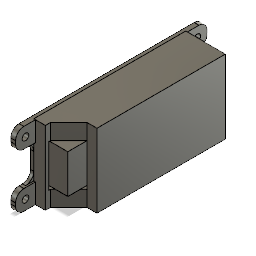
Kanssi_v2 (Autodesk Fusion 360 design; units mm, degrees)
Autodesk Fusion 360 part; units mm, degrees
sketch "PCB" plane through (0, 0, 0) normal (1, 0, 0) x (0, 0, -1)
  line L0 (0, 0) -> (-84.582, 0)
  line L1 (-84.582, 0) -> (-84.582, 37.465)
  line L2 (-84.582, 37.465) -> (0, 37.465)
  line L3 (0, 37.465) -> (0, 0)
  circle A0 centre (-78.867, 3.175) radius 1.55
  circle A1 centre (-3.683, 3.175) radius 1.55
  circle A2 centre (-78.867, 34.29) radius 1.55
  circle A3 centre (-3.683, 34.29) radius 1.55
  dimension "d1" = 37.465
  dimension "d2" = 84.582
  dimension "d3" = 3.1
  dimension "d4" = 75.184
  dimension "d5" = 3.1
  dimension "d7" = 31.115
  dimension "d10" = 5.715
  dimension "d11" = 3.175
  dimension "d12" = 3.1
  dimension "d242" = 3.1
  constraint horizontal L0
  constraint vertical L1
  constraint horizontal L2
  constraint vertical L3
  constraint coincident L0.start L3.end
  measures "d1" distance of L0.start L2.end
  measures "d2" distance of L0.start L0.end
  measures "d3" diameter of A1
  measures "d4" distance of A0.centre A1.centre
  measures "d5" diameter of A2
  measures "d7" distance of A0.centre A2.centre
  measures "d10" distance of L1 A0.centre
  measures "d11" distance of L0 A0.centre
  measures "d12" diameter of A3
  measures "d242" diameter of A0
extrude "Extrude1" add sketch "PCB" along normal blind 2 makes body 1
sketch "Komponentit" plane through (2, 0, 0) normal (1, 0, 0) x (0, 0, -1)
  circle A0 centre (-3.683, 3.175) radius 1.55
  circle A1 centre (-78.867, 34.29) radius 1.55
  circle A2 centre (-78.867, 3.175) radius 1.55
  circle A3 centre (-3.683, 34.29) radius 1.55
  line L0 (0, 37.465) -> (-84.582, 37.465)
  line L1 (-84.582, 37.465) -> (-84.582, 0)
  line L2 (-84.582, 0) -> (0, 0)
  line L3 (0, 0) -> (0, 37.465)
  line L4 (-44.958, 11.557) -> (-70.358, 11.557)
  line L5 (-70.358, 36.957) -> (-44.958, 36.957)
  line L6 (-70.358, 36.957) -> (-44.958, 36.957)
  line L7 (-44.958, 36.957) -> (-44.958, 11.557)
  line L8 (-44.958, 11.557) -> (-70.358, 11.557)
  line L9 (-70.358, 11.557) -> (-70.358, 36.957)
  line L10 (-84.582, 37.465) -> (0, 37.465)
  line L11 (0, 37.465) -> (0, 0)
  line L12 (0, 0) -> (-84.582, 0)
  line L13 (-84.582, 0) -> (-84.582, 37.465)
  line L14 (-70.358, 11.1514) -> (-44.9504, 11.1514)
  line L15 (-44.9504, 11.1514) -> (-44.9504, 0.635)
  line L16 (-44.9504, 0.635) -> (-70.358, 0.635)
  line L17 (-70.358, 0.635) -> (-70.358, 11.1514)
  line L18 (-44.5991, 24) -> (-22.6991, 24)
  line L19 (-22.6991, 24) -> (-22.6991, 1.1)
  line L20 (-22.6991, 1.1) -> (-44.5991, 1.1)
  line L21 (-44.5991, 1.1) -> (-44.5991, 24)
  line L22 (-84.582, 30.48) -> (-71, 30.48)
  line L23 (-71, 30.48) -> (-71, 7.112)
  line L24 (-71, 7.112) -> (-84.582, 7.112)
  line L25 (-84.582, 7.112) -> (-84.582, 30.48)
  line L26 (0, 37.465) -> (-28, 37.465)
  line L27 (0, 37.465) -> (-21, 37.465)
  line L28 (-28, 37.465) -> (-21, 37.465)
  line L29 (-21, 37.465) -> (-21, 26.465)
  line L30 (-21, 26.465) -> (-28, 26.465)
  line L31 (-28, 26.465) -> (-28, 37.465)
  dimension "d22" = 25.4
  dimension "d23" = 14.224
  dimension "d24" = 0.508
  dimension "d25" = 25.4
  dimension "d26" = 10.5164
  dimension "d27" = 25.4076
  dimension "d28" = 0.635
  dimension "d29" = 14.224
  dimension "d30" = 21.9
  dimension "d31" = 22.9
  dimension "d33" = 1.1
  dimension "d34" = 0.3589
  dimension "d41" = 7.112
  dimension "d42" = 6.985
  dimension "d43" = 0.642
  dimension "d355" = 28
  dimension "d356" = 21
  dimension "d357" = 11
  constraint horizontal L4
  constraint horizontal L6
  constraint vertical L7
  constraint horizontal L8
  constraint vertical L9
  constraint horizontal L10
  constraint vertical L11
  constraint horizontal L12
  constraint vertical L13
  constraint coincident L2.end L3.start
  constraint coincident L0.end L1.start
  constraint horizontal L14
  constraint vertical L15
  constraint horizontal L16
  constraint vertical L17
  constraint horizontal L18
  constraint vertical L19
  constraint horizontal L20
  constraint vertical L21
  constraint horizontal L22
  constraint vertical L23
  constraint horizontal L24
  constraint vertical L25
  constraint coincident L1 L22.start
  constraint coincident L0.start L3.end
  constraint perpendicular L3 L26
  constraint perpendicular L11 L27
  constraint horizontal L28
  constraint vertical L29
  constraint horizontal L30
  constraint vertical L31
  measures "d22" distance of L4 L5
  measures "d23" distance of L9 L13
  measures "d24" distance of L6 L10
  measures "d25" distance of L7 L9
  measures "d26" distance of L14.start L16.end
  measures "d27" distance of L15 L17
  measures "d28" distance of L12 L16
  measures "d29" distance of L13 L17
  measures "d30" distance of L19 L21
  measures "d31" distance of L18 L20
  measures "d33" distance of L12 L20
  measures "d34" distance of L7 L21
  measures "d41" distance of L12 L24
  measures "d42" distance of L10 L22
  measures "d43" distance of L9 L23
  measures "d355" distance of L0.start L26.end
  measures "d356" distance of L0.start L27.end
  measures "d357" distance of L26.end L30.end
extrude "Extrude4" add sketch "Komponentit" along normal blind 15 contours L18 L19 L20 L21 bodies 1
extrude "Extrude3" add sketch "Komponentit" along normal blind 15.8 contours L14 L15 L16 L17 bodies 1
extrude "Extrude2" add sketch "Komponentit" along normal blind 16.3 contours L4 L5 L6 L7 L8 L9 bodies 1
sketch "Sketch7" plane through (2, 0, 0) normal (1, 0, 0) x (0, 0, -1)
  line L0 (-70.358, 11.557) -> (-70.358, 36.957)
  line L1 (-70.358, 36.957) -> (-44.958, 36.957)
  line L2 (-44.958, 36.957) -> (-44.958, 11.557)
  line L3 (-44.958, 11.557) -> (-70.358, 11.557)
  line L4 (-70.358, 0.635) -> (-70.358, 11.1514)
  line L5 (-70.358, 11.1514) -> (-44.9504, 11.1514)
  line L6 (-44.9504, 11.1514) -> (-44.9504, 0.635)
  line L7 (-44.9504, 0.635) -> (-70.358, 0.635)
  line L8 (-44.5991, 1.1) -> (-44.5991, 24)
  line L9 (-44.5991, 24) -> (-22.6991, 24)
  line L10 (-22.6991, 24) -> (-22.6991, 1.1)
  line L11 (-22.6991, 1.1) -> (-44.5991, 1.1)
  line L12 (-84.582, 0) -> (0, 0)
  line L13 (0, 0) -> (0, 37.465)
  line L14 (0, 37.465) -> (-84.582, 37.465)
  line L15 (-84.582, 37.465) -> (-84.582, 0)
  circle A0 centre (-3.683, 34.29) radius 1.55
  circle A1 centre (-78.867, 3.175) radius 1.55
  circle A2 centre (-78.867, 34.29) radius 1.55
  circle A3 centre (-3.683, 3.175) radius 1.55
  line L16 (25, -5) -> (50, -5)
  line L17 (50, -5) -> (50, -30)
  line L18 (50, -30) -> (25, -30)
  line L19 (25, -30) -> (25, -5)
  circle A4 centre (37.5, -17.5) radius 12.5
  line L20 (25, -30) -> (50, -30)
  line L21 (50, -30) -> (50, -34)
  line L22 (50, -34) -> (25, -34)
  line L23 (25, -34) -> (25, -30)
  circle A5 centre (37.5, -17.5) radius 3
  dimension "d111" = 25
  dimension "d112" = 25
  dimension "d113" = 25
  dimension "d114" = 4
  dimension "d115" = 25
  dimension "d118" = 6
  constraint horizontal L16
  constraint vertical L17
  constraint horizontal L18
  constraint vertical L19
  constraint horizontal L20
  constraint vertical L21
  constraint horizontal L22
  constraint vertical L23
  constraint concentric A4 A5
  measures "d111" distance of L16.start L16.end
  measures "d112" distance of L16.start L18.end
  measures "d113" distance of L18.end L17.end
  measures "d114" distance of L18.end L22.end
  measures "d115" diameter of A4
  measures "d118" diameter of A5
extrude "Extrude6" add sketch "Sketch7" along normal blind 12 separate body contours A4 | L18 L19 A4 L20 | L17 L18 A4 L20 | L18 L20 L21 L22 L23 makes body 2
extrude "Extrude8" add sketch "Komponentit" along normal blind 13 contours L1 L13 L22 L23 L24 L25 bodies 1
sketch "Sketch1" plane through (0, 0, 0) normal (-1, 0, 0) x (0, 0, 1) in component "Component"
  line L0 (84.582, 37.465) -> (0, 37.465)
  line L1 (0, 37.465) -> (0, 0)
  line L2 (0, 0) -> (84.582, 0)
  line L3 (84.582, 0) -> (84.582, 37.465)
  line L4 (-1.5, 38.965) -> (86.082, 38.965)
  line L5 (86.082, 38.965) -> (86.082, -1.5)
  line L6 (86.082, -1.5) -> (-1.5, -1.5)
  line L7 (-1.5, -1.5) -> (-1.5, 38.965)
  line L8 (88.082, -3.5) -> (-3.5, -3.5)
  line L9 (-3.5, -3.5) -> (-3.5, 40.965)
  line L10 (-3.5, 40.965) -> (88.082, 40.965)
  line L11 (88.082, 40.965) -> (88.082, -3.5)
  line L12 (71, 30.48) -> (71, 7.112)
  circle A0 centre (78.867, 34.29) radius 2.1
  circle A1 centre (3.683, 34.29) radius 2.1
  circle A2 centre (3.683, 3.175) radius 2.1
  circle A3 centre (78.867, 3.175) radius 2.1
  circle A4 centre (3.683, 34.29) radius 0.9
  circle A5 centre (3.683, 3.175) radius 1.05
  circle A6 centre (78.867, 34.29) radius 1.05
  circle A7 centre (78.867, 3.175) radius 1.05
  circle A8 centre (3.683, 3.175) radius 3
  circle A9 centre (3.683, 34.29) radius 3
  circle A10 centre (78.867, 34.29) radius 3
  circle A11 centre (78.867, 3.175) radius 3
  dimension "d243" = 1.5
  dimension "d244" = 1.5
  dimension "d245" = 1.5
  dimension "d246" = 1.5
  dimension "d247" = -2
  dimension "d250" = 4.2
  dimension "d251" = 4.2
  dimension "d252" = 4.2
  dimension "d253" = 4.2
  dimension "d254" = 1.8
  dimension "d347" = 2.1
  dimension "d348" = 2.1
  dimension "d349" = 2.1
  dimension "d350" = 6
  dimension "d351" = 6
  dimension "d352" = 6
  dimension "d353" = 6
  constraint horizontal L4
  constraint vertical L5
  constraint horizontal L6
  constraint vertical L7
  constraint concentric A1 A4
  constraint concentric A2 A5
  constraint concentric A5 A8
  constraint concentric A1 A9
  constraint concentric A6 A10
  constraint concentric A3 A11
  measures "d243" distance of L0 L4
  measures "d244" distance of L1 L7
  measures "d245" distance of L2 L6
  measures "d246" distance of L3 L5
  measures "d250" diameter of A0
  measures "d251" diameter of A1
  measures "d252" diameter of A2
  measures "d253" diameter of A3
  measures "d254" diameter of A4
  measures "d347" diameter of A5
  measures "d348" diameter of A6
  measures "d349" diameter of A7
  measures "d350" diameter of A8
  measures "d351" diameter of A9
  measures "d352" diameter of A10
  measures "d353" diameter of A11
extrude "Extrude1'" add sketch "Sketch1" along normal blind 2 separate body contours L0 L1 L2 L3 | L4 L5 L6 L7 | L8 L9 L10 L11 | A1 | A4 | A8 | A9 | A10 | A11 makes body 3 in component "Component"
move_body "Move3" bodies 1 to x (1, 0, 0) y (0, 1, 0) z (0, 0, 1) at (2, 0, 0)
extrude "Extrude2'" add sketch "Sketch1" against normal blind 2 contours A0 | A1 | A2 | A3 | A4 | A8 | A9 | A10 | A11 bodies 3 in component "Component"
extrude "Extrude3'" add sketch "Sketch1" against normal blind 4 contours A4 bodies 3 in component "Component"
extrude "Extrude1''" add sketch "Sketch1" against normal blind 22 separate body contours L8 L9 L10 L11 makes body 4 in component "Component'"
sketch "Sketch1 (2)" plane through (22, 0, 0) normal (1, 0, 0) x (0, 0, -1) in component "Component'"
  line L0 (1.5, -1.5) -> (-86.082, -1.5)
  line L1 (-86.082, -1.5) -> (-86.082, 38.965)
  line L2 (-86.082, 38.965) -> (1.5, 38.965)
  line L3 (1.5, 38.965) -> (1.5, -1.5)
  line L4 (3.5, 40.965) -> (-88.082, 40.965)
  line L5 (-88.082, 40.965) -> (-88.082, -3.5)
  line L6 (-88.082, -3.5) -> (3.5, -3.5)
  line L7 (3.5, -3.5) -> (3.5, 40.965)
  line L8 (1.5, -1.5) -> (-8.866, -1.5)
  line L9 (-8.866, -1.5) -> (-8.866, 7.85)
  line L10 (-8.866, 7.85) -> (1.5, 7.85)
  line L11 (1.5, 7.85) -> (1.5, -1.5)
  line L12 (1.5, -1.5) -> (-8.866, 7.85) construction
  line L13 (-8.866, -1.5) -> (1.5, 7.85) construction
  line L14 (-72.0095, 40.965) -> (-72.0095, -3.5)
  circle A0 centre (-3.683, 3.175) radius 1.05
  circle A1 centre (-78.867, 34.29) radius 1.05
  circle A2 centre (-78.867, 3.175) radius 1.05
  point P0 (-3.683, 34.29)
  point P1 (-3.683, 34.29)
  point P2 (-3.683, 3.175)
  point P3 (-78.867, 3.175)
  point P4 (-78.867, 34.29)
  point P5 (-3.683, 3.175)
  dimension "d264" = 2.1
  dimension "d337" = 2.1
  dimension "d338" = 2.1
  constraint coincident P1 P0
  constraint perpendicular L8 L9
  constraint parallel L8 L10
  constraint parallel L9 L11
  constraint horizontal L8
  constraint coincident L0.start L3.end
  constraint coincident L12 P5
  constraint coincident L13 P5
  constraint coincident P5 P2
  constraint coincident L4 L14.start
  constraint coincident L6 L14.end
  constraint perpendicular L6 L14
  constraint coincident P4 A1.centre
  constraint coincident P3 A2.centre
  measures "d264" diameter of A0
  measures "d337" diameter of A1
  measures "d338" diameter of A2
extrude "Extrude2''" add sketch "Sketch1 (2)" against normal blind 17 contours L0 L2 L3 L4 L6 L7 L8 L11 L14 | L0 L3 L8 L9 L10 L11 bodies 4 in component "Component'"
extrude "Extrude3''" cut sketch "Sketch1 (2)" against normal blind 13 contours A0 bodies 4 in component "Component'"
extrude "Extrude4'" add sketch "Sketch1 (2)" along normal blind 2 contours L0 L2 L3 L4 L6 L7 L8 L11 L14 | L0 L3 L8 L9 L10 L11 | L0 L2 L3 L9 L10 L14 | A0 bodies 4 in component "Component'"
extrude "Extrude5" cut sketch "Sketch1 (2)" against normal blind 18 contours L0 L1 L2 L4 L5 L6 L14 bodies 4 in component "Component'"
sketch "Sketch2" plane through (0, 0, 72.0095) normal (0, 0, 1) x (1, 0, 0) in component "Component'"
  line L0 (22, -1.5) -> (4, -1.5)
  line L1 (4, -1.5) -> (4, -3.5)
  line L2 (4, -3.5) -> (24, -3.5)
  line L3 (24, -3.5) -> (24, 40.965)
  line L4 (24, 40.965) -> (4, 40.965)
  line L5 (4, 40.965) -> (4, 38.965)
  line L6 (4, 38.965) -> (22, 38.965)
  line L7 (4, 40.965) -> (24, 40.965)
  line L8 (24, 40.965) -> (24, -3.5)
  line L9 (24, -3.5) -> (4, -3.5)
  line L10 (4, -3.5) -> (4, 40.965)
  line L11 (4, 40.965) -> (5, 40.965)
  line L12 (4, 31.48) -> (18, 31.48)
  line L13 (18, 31.48) -> (18, 6.112)
  line L14 (18, 6.112) -> (4, 6.112)
  line L15 (4, 30.48) -> (17, 30.48)
  line L16 (17, 30.48) -> (17, 7.112)
  line L17 (4, 7.112) -> (17, 7.112)
  line L18 (5, 40.965) -> (5, 31.48)
  line L19 (4, -3.5) -> (5, -3.5)
  line L20 (5, -3.5) -> (5, 6.112)
  line L21 (5, 40.965) -> (7, 40.965)
  line L22 (7, 40.965) -> (7, 31.48)
  line L23 (7, 31.48) -> (5, 31.48)
  line L24 (5, 31.48) -> (5, 40.965)
  line L25 (5, 6.112) -> (7, 6.112)
  line L26 (7, 6.112) -> (7, -3.5)
  line L27 (7, -3.5) -> (5, -3.5)
  line L28 (5, -3.5) -> (5, 6.112)
  line L29 (22, 38.965) -> (22, -1.5)
  dimension "d271" = 1
  dimension "d272" = 1
  dimension "d273" = 1
  dimension "d274" = 1
  dimension "d275" = 1
  dimension "d278" = 2
  dimension "d279" = 2
  constraint horizontal L7
  constraint vertical L8
  constraint horizontal L9
  constraint vertical L10
  constraint coincident L2.end L3.start
  constraint coincident L4.end L5.start
  constraint perpendicular L10 L11
  constraint coincident L10 L12.start
  constraint perpendicular L10 L12
  constraint perpendicular L12 L13
  constraint coincident L10 L14.end
  constraint perpendicular L10 L14
  constraint coincident L12 L18.end
  constraint perpendicular L12 L18
  constraint coincident L1.end L2.start
  constraint perpendicular L1 L19
  constraint coincident L14 L20.end
  constraint perpendicular L14 L20
  constraint horizontal L21
  constraint vertical L22
  constraint horizontal L23
  constraint vertical L24
  constraint coincident L12 L22.end
  constraint horizontal L25
  constraint vertical L26
  constraint horizontal L27
  constraint vertical L28
  measures "d271" distance of L4.end L11.end
  measures "d272" distance of L12 L15
  measures "d273" distance of L13 L16
  measures "d274" distance of L14 L17
  measures "d275" distance of L1.end L19.end
  measures "d278" distance of L11.end L21.end
  measures "d279" distance of L20.end L25.end
extrude "Extrude6'" add sketch "Sketch2" along normal blind 2 contours L0 L2 L3 L4 L6 L7 L8 L9 L22 L26 L29 | L0 L6 L12 L13 L14 L22 L26 L29 | L0 L2 L9 L20 L26 L27 L28 | L0 L14 L20 L25 L26 L28 | L0 L1 L2 L9 L10 L19 L20 L28 | L6 L12 L18 L22 L23 L24 | L4 L6 L7 L18 L21 L22 L24 | L4 L5 L6 L7 L10 L11 L18 L24 bodies 4 in component "Component'"
extrude "Extrude7" add sketch "Sketch2" along normal blind 16.072 contours L0 L2 L9 L20 L26 L27 L28 | L0 L14 L20 L25 L26 L28 | L0 L1 L2 L9 L10 L19 L20 L28 | L6 L12 L18 L22 L23 L24 | L4 L6 L7 L18 L21 L22 L24 | L4 L5 L6 L7 L10 L11 L18 L24 bodies 4 in component "Component'"
sketch "Sketch3" plane through (0, 0, 88.082) normal (0, 0, 1) x (1, 0, 0) in component "Component'"
  line L0 (4, -3.5) -> (4, 40.965)
  line L1 (4, 40.965) -> (0, 40.965)
  line L2 (0, 40.965) -> (0, -3.5)
  line L3 (0, -3.5) -> (4, -3.5)
  line L4 (0, 40.965) -> (7, 40.965)
  line L5 (7, 40.965) -> (7, -3.5)
  line L6 (7, -3.5) -> (0, -3.5)
  line L7 (0, -3.5) -> (0, 40.965)
  constraint horizontal L4
  constraint vertical L5
  constraint horizontal L6
  constraint vertical L7
  constraint coincident L1.end L2.start
extrude "Extrude8'" add sketch "Sketch3" against normal blind 2 bodies 4 in component "Component'"
sketch "Sketch4" plane through (7, 0, 0) normal (1, 0, 0) x (0, 0, -1) in component "Component'"
  line L0 (-88.082, -3.5) -> (-74.0095, -3.5)
  line L1 (-74.0095, -3.5) -> (-74.0095, 6.112)
  line L2 (-74.0095, 6.112) -> (-86.082, 6.112)
  line L3 (-86.082, 6.112) -> (-86.082, 31.48)
  line L4 (-86.082, 31.48) -> (-74.0095, 31.48)
  line L5 (-74.0095, 31.48) -> (-74.0095, 40.965)
  line L6 (-74.0095, 40.965) -> (-88.082, 40.965)
  line L7 (-88.082, 40.965) -> (-88.082, -3.5)
  circle A0 centre (-78.867, 34.29) radius 1.55
  circle A1 centre (-78.867, 3.175) radius 1.55
  point P0 (-78.867, 3.175)
  point P1 (-78.867, 34.29)
  dimension "d284" = 3.1
  dimension "d285" = 3.1
  constraint coincident P1 A0.centre
  constraint coincident P0 A1.centre
  measures "d284" diameter of A0
  measures "d285" diameter of A1
sketch "Sketch2 (2)" plane through (-2, 0, 0) normal (-1, 0, 0) x (0, 0, 1) in component "Component"
  line L0 (88.082, 40.965) -> (-3.5, 40.965)
  line L1 (-3.5, 40.965) -> (-3.5, -3.5)
  line L2 (-3.5, -3.5) -> (88.082, -3.5)
  line L3 (88.082, -3.5) -> (88.082, 40.965)
  line L4 (-3.5, 40.965) -> (-15.5, 40.965)
  line L5 (-15.5, 40.965) -> (-15.5, -3.5)
  line L6 (-15.5, -3.5) -> (-3.5, -3.5)
  line L7 (-3.5, -3.5) -> (-3.5, 40.965)
  circle A0 centre (-9.5, 34.965) radius 2
  circle A1 centre (-9.5, 2.5) radius 2
  line L8 (-15.5, 28.965) -> (-3.5, 28.965)
  line L9 (-3.5, 28.965) -> (-3.5, 8.5)
  line L10 (-3.5, 8.5) -> (-15.5, 8.5)
  line L11 (-15.5, 8.5) -> (-15.5, 28.965)
  line L12 (88.082, 40.965) -> (100.082, 40.965)
  line L13 (100.082, 40.965) -> (100.082, -3.5)
  line L14 (100.082, -3.5) -> (88.082, -3.5)
  line L15 (88.082, -3.5) -> (88.082, 40.965)
  circle A2 centre (94.082, 34.965) radius 2
  circle A3 centre (94.082, 2.5) radius 2
  line L16 (88.082, 28.965) -> (100.082, 28.965)
  line L17 (88.082, 8.5) -> (100.082, 8.5)
  line L18 (7.183, -0.325) -> (0.183, -0.325)
  line L19 (0.183, -0.325) -> (0.183, 6.675)
  line L20 (0.183, 6.675) -> (7.183, 6.675)
  line L21 (7.183, 6.675) -> (7.183, -0.325)
  line L22 (7.183, -0.325) -> (0.183, 6.675) construction
  line L23 (0.183, -0.325) -> (7.183, 6.675) construction
  line L24 (82.367, -0.325) -> (75.367, -0.325)
  line L25 (75.367, -0.325) -> (75.367, 6.675)
  line L26 (75.367, 6.675) -> (82.367, 6.675)
  line L27 (82.367, 6.675) -> (82.367, -0.325)
  line L28 (82.367, -0.325) -> (75.367, 6.675) construction
  line L29 (75.367, -0.325) -> (82.367, 6.675) construction
  line L30 (75.367, 30.79) -> (82.367, 30.79)
  line L31 (82.367, 30.79) -> (82.367, 37.79)
  line L32 (82.367, 37.79) -> (75.367, 37.79)
  line L33 (75.367, 37.79) -> (75.367, 30.79)
  line L34 (75.367, 30.79) -> (82.367, 37.79) construction
  line L35 (82.367, 30.79) -> (75.367, 37.79) construction
  circle A4 centre (78.867, 3.175) radius 2.1
  circle A5 centre (78.867, 34.29) radius 2.1
  circle A6 centre (3.683, 3.175) radius 2.1
  circle A7 centre (78.867, 34.29) radius 2.1
  circle A8 centre (3.683, 3.175) radius 2.1
  circle A9 centre (78.867, 3.175) radius 2.1
  point P0 (3.683, 3.175)
  point P1 (78.867, 3.175)
  point P2 (78.867, 34.29)
  dimension "d301" = 12
  dimension "d302" = 4
  dimension "d303" = 4
  dimension "d304" = 6
  dimension "d305" = 6
  dimension "d306" = 6
  dimension "d307" = 6
  dimension "d308" = 6
  dimension "d309" = 6
  dimension "d310" = 12
  dimension "d311" = 4
  dimension "d312" = 4
  dimension "d313" = 6
  dimension "d314" = 6
  dimension "d315" = 6
  dimension "d316" = 6
  dimension "d317" = 44.465
  dimension "d318" = 44.465
  dimension "d319" = 20.465
  dimension "d320" = 12
  dimension "d324" = 7
  dimension "d325" = 7
  dimension "d326" = 7
  dimension "d327" = 7
  dimension "d328" = 7
  dimension "d329" = 7
  dimension "d330" = 4.2
  dimension "d331" = 4.2
  dimension "d332" = 4.2
  constraint horizontal L4
  constraint vertical L5
  constraint horizontal L6
  constraint vertical L7
  constraint coincident L0.end L1.start
  constraint horizontal L8
  constraint vertical L9
  constraint horizontal L10
  constraint vertical L11
  constraint coincident L7 L9.end
  constraint coincident L5 L8.start
  constraint horizontal L12
  constraint vertical L13
  constraint horizontal L14
  constraint vertical L15
  constraint coincident L0.start L3.end
  constraint coincident L15 L16.start
  constraint coincident L13 L16.end
  constraint perpendicular L13 L16
  constraint coincident L15 L17.start
  constraint coincident L13 L17.end
  constraint perpendicular L13 L17
  constraint perpendicular L18 L19
  constraint parallel L18 L20
  constraint parallel L19 L21
  constraint horizontal L18
  constraint coincident L22 P0
  constraint coincident L23 P0
  constraint perpendicular L24 L25
  constraint parallel L24 L26
  constraint parallel L25 L27
  constraint horizontal L24
  constraint coincident L28 P1
  constraint coincident L29 P1
  constraint perpendicular L30 L31
  constraint parallel L30 L32
  constraint parallel L31 L33
  constraint horizontal L30
  constraint coincident L34 P2
  constraint coincident L35 P2
  constraint coincident P2 A5.centre
  measures "d301" distance of L0.end L4.end
  measures "d302" diameter of A0
  measures "d303" diameter of A1
  measures "d304" distance of L4 A0.centre
  measures "d305" distance of L6 A1.centre
  measures "d306" distance of L7 A0.centre
  measures "d307" distance of L7 A1.centre
  measures "d308" distance of A0.centre L8
  measures "d309" distance of A1.centre L10
  measures "d310" distance of L0.start L12.end
  measures "d311" diameter of A2
  measures "d312" diameter of A3
  measures "d313" distance of L12 A2.centre
  measures "d314" distance of L14 A3.centre
  measures "d315" distance of L15 A3.centre
  measures "d316" distance of L15 A2.centre
  measures "d317" distance of L4 L6
  measures "d318" distance of L12 L14
  measures "d319" distance of L16 L17
  measures "d320" distance of L12 L16
  measures "d324" distance of L19.end L20.end
  measures "d325" distance of L18.end L19.end
  measures "d326" distance of L25.end L26.end
  measures "d327" distance of L24.end L25.end
  measures "d328" distance of L31.end L32.end
  measures "d329" distance of L30.end L31.end
  measures "d330" diameter of A4
  measures "d331" diameter of A5
  measures "d332" diameter of A6
extrude "Extrude4''" add sketch "Sketch2 (2)" against normal blind 3 contours L3 L12 L13 L15 L16 | L1 L4 L5 L7 L8 | L3 L13 L14 L15 L17 | L1 L5 L6 L7 L10 bodies 3 in component "Component"
fillet "Fillet2" radius 5 12 edges at (-1, 8.5, -3.5) (-0.5, 8.5, -15.5) (-0.5, -3.5, -15.5) (-1, 28.965, -3.5) (-0.5, 28.965, -15.5) (-0.5, 40.965, -15.5) (-0.5, 40.965, 100.082) (-0.5, 28.965, 100.082) (-0.5, 8.5, 100.082) (-1, 8.5, 88.082) (-0.5, -3.5, 100.082) (-1, 28.965, 88.082) on bodies 3 in component "Component"
extrude "Extrude5'" cut sketch "Sketch2 (2)" against normal blind 2 contours A4 A9 | A5 A7 | A6 A8 bodies 3 in component "Component"
chamfer "Chamfer2" distance 11 angle 45 2 edges at (7, 36.2225, 74.0095) (7, 1.306, 74.0095) on bodies 4 in component "Component'"
extrude "Extrude10" cut sketch "Sketch1 (2)" along normal blind -12 and the other way blind 17 contours A1 | A2 bodies 4 in component "Component'"
chamfer "Chamfer2'" distance 1.2 angle 45 4 edges at (0, 33.2052, 0.886) (0, 2.0902, 0.886) (0, 33.2052, 76.07) (0, 2.0902, 76.07) on bodies 3 in component "Component"
sketch "Sketch5" plane through (24, 0, 0) normal (1, 0, 0) x (0, 0, -1) in component "Component'"
  line L0 (-74.0095, -3.5) -> (3.5, -3.5)
  line L1 (3.5, -3.5) -> (3.5, 40.965)
  line L2 (3.5, 40.965) -> (-74.0095, 40.965)
  line L3 (-74.0095, 40.965) -> (-74.0095, -3.5)
  line L4 (-21, 37.465) -> (-28, 37.465)
  line L5 (-28, 37.465) -> (-28, 26.465)
  line L6 (-28, 26.465) -> (-21, 26.465)
  line L7 (-21, 26.465) -> (-21, 37.465)
  line L8 (-28, 37.465) -> (-21, 37.465)
  line L9 (-21, 37.465) -> (-21, 31.465)
  line L10 (-21, 31.465) -> (-28, 31.465)
  line L11 (-28, 31.465) -> (-28, 37.465)
  line L12 (-24.5, 37.465) -> (-24.5, 31.465)
  line L13 (-25, 37.465) -> (-25, 31.465)
  line L14 (-24, 37.465) -> (-24, 31.465)
  line L15 (-21, 31.965) -> (-28, 31.965)
  line L16 (-21, 30.965) -> (-28, 30.965)
  line L17 (-21, 40.965) -> (-28, 40.965)
  line L18 (-28, 40.965) -> (-28, 26.465)
  line L19 (-28, 26.465) -> (-21, 26.465)
  line L20 (-21, 26.465) -> (-21, 40.965)
  line L21 (-19, 40.965) -> (-30, 40.965)
  line L22 (-30, 40.965) -> (-30, 24.465)
  line L23 (-30, 24.465) -> (-19, 24.465)
  line L24 (-19, 24.465) -> (-19, 40.965)
  line L25 (-19, 26.465) -> (-30, 26.465)
  point P0 (-21, 37.465)
  point P1 (-28, 26.465)
  dimension "d358" = 6
  dimension "d359" = 0.5
  dimension "d360" = -0.5
  dimension "d361" = 0.5
  dimension "d362" = -0.5
  dimension "d369" = 2
  dimension "d370" = 2
  dimension "d371" = 2
  constraint horizontal L4
  constraint vertical L5
  constraint horizontal L6
  constraint vertical L7
  constraint coincident P1 L5.end
  constraint coincident P0 L4.start
  constraint horizontal L8
  constraint vertical L9
  constraint horizontal L10
  constraint vertical L11
  constraint midpoint L4 L12.start
  constraint midpoint L10 L12.end
  constraint perpendicular L10 L12
  constraint horizontal L17
  constraint vertical L18
  constraint horizontal L19
  constraint vertical L20
  constraint coincident L2 L17.start
  constraint horizontal L21
  constraint vertical L22
  constraint horizontal L23
  constraint vertical L24
  constraint coincident L2 L21.start
  constraint coincident L24 L25.start
  constraint coincident L22 L25.end
  constraint perpendicular L22 L25
  measures "d358" distance of L4.end L10.end
  measures "d369" distance of L9 L24
  measures "d370" distance of L11 L22
  measures "d371" distance of L19 L23
component "Component" placed x (1, 0, 0) y (0, 1, 0) z (0, 0, 1) at (0, 0, 0)
component "Component'" placed x (1, 0, 0) y (0, 1, 0) z (0, 0, 1) at (0, 0, 0)
hidden bodies 2
